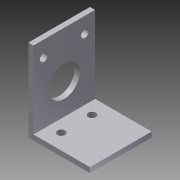
# Autodesk Inventor part: Angle Aluminum P60 Mount
Saved by Autodesk Inventor 2013 (Build 170138000, 138)
## iProperties
Created: 2013-03-11
Part Number: Angle Aluminum P60 Mount
Material: Aluminum 6061
Document SubType Name: Modeling
Designer: Moses
Mass: 27.796 g
Surface Area: 73.4229 cm^2
Volume: 10.2568 cm^3
Density: 2.71 g/cm^3
Author: Moses
Autodesk Inventor part; units mm, degrees
ref_plane "YZ Plane" through (0, 0, 0) normal (1, 0, 0) x (0, 1, 0)
ref_plane "XZ Plane" through (0, 0, 0) normal (0, 1, 0) x (-1, 0, 0)
ref_plane "XY Plane" through (0, 0, 0) normal (0, 0, 1) x (1, 0, 0)
sketch "Sketch1" plane through (0, 0, 0) normal (0, 0, 1) x (1, 0, 0)
  line L0 (0, 0) -> (38.1, 0)
  line L1 (0, 0) -> (0, 50.8)
  line L2 (0, 50.8) -> (3.175, 50.8)
  line L3 (3.175, 50.8) -> (3.175, 3.175)
  line L4 (3.175, 3.175) -> (38.1, 3.175)
  line L5 (38.1, 3.175) -> (38.1, 0)
  dimension "d0" = 38.1
  dimension "d1" = 50.8
  dimension "d2" = 3.175
  constraints: 12 end point, 4 perpendicular, 2 parallel, 1 horizontal
  measures "d0" distance of L0.start L0.end
  measures "d1" distance of L0.start L1.end
  measures "d2" distance of L1.end L2.end
extrude "Extrusion1" add sketch "Sketch1" along normal blind 38.1
sketch "Sketch2" plane through (0, 0, 0) normal (-1, 0, 0) x (0, 0, 1)
  line L0 (0, 0) -> (38.1, 0) projected
  line L1 (0, 50.8) -> (38.1, 50.8) projected
  line L2 (19.05, 50.8) -> (19.05, 0) construction
  line L3 (6.35, 41.275) -> (31.75, 41.275) construction
  circle A0 centre (6.35, 41.275) radius 2.3812
  circle A1 centre (31.75, 41.275) radius 2.3813
  circle A2 centre (19.05, 22.225) radius 9.525
  point P0 (19.05, 41.275)
  dimension "d5" = 25.4
  dimension "d6" = 9.525
  dimension "d7" = 4.7625
  dimension "d8" = 4.7625
  dimension "d11" = 19.05
  dimension "d12" = 22.225
  constraints: 4 end point, 3 centre point, 3 midpoint, 2 coincident, 2 point on line, 1 perpendicular
  measures "d5" distance of L3.start L3.end
  measures "d6" distance between parallel lines of L3 L1
  measures "d7" diameter of A0
  measures "d8" diameter of A1
  measures "d11" diameter of A2
  measures "d12" distance from line of L0 A2.centre
extrude "Extrusion2" cut sketch "Sketch2" against normal blind 38.1
sketch "Sketch3" plane through (0, 0, 0) normal (0, -1, 0) x (1, 0, 0)
  line L0 (38.1, 0) -> (38.1, 38.1) projected
  line L1 (0, 0) -> (0, 38.1) projected
  circle A0 centre (10.795, 28.575) radius 2.3813
  line L2 (10.795, 28.575) -> (10.795, 9.525) construction
  circle A1 centre (10.795, 9.525) radius 2.3813
  line L3 (0, 19.05) -> (38.1, 19.05) construction
  point P0 (10.795, 19.05)
  dimension "d13" = 19.05
  dimension "d17" = 4.7625
  dimension "d18" = 10.795
  constraints: 4 end point, 3 midpoint, 2 centre point, 1 coincident, 1 equal radius, 1 parallel, 1 point on line
  measures "d13" distance of L2.start L2.end
  measures "d17" diameter of A0
  measures "d18" distance between parallel lines of L2 L1
extrude "Extrusion3" cut sketch "Sketch3" against normal blind 25.4
body "Solid1"
